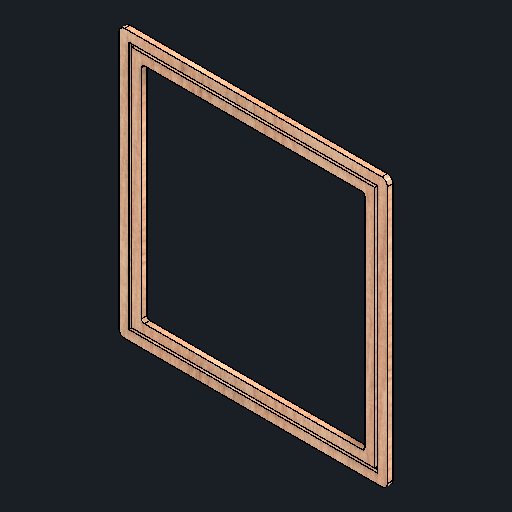
# Autodesk Inventor part: Part1
Saved by Autodesk Inventor 2026.2 (Build 302298000, 298)
## iProperties
Created: 2026-06-15
Part Number: Part1
Material: Wood (Birch)
Document SubType Name: Modeling
Designer: JoshuaEah
Density: 0.55 g/cm^3
Appearance: Birch - Natural Polished
Author: JoshuaEah
Autodesk Inventor part; units mm, degrees
ref_plane "YZ Plane" through (0, 0, 0) normal (1, 0, 0) x (0, 1, 0)
ref_plane "XZ Plane" through (0, 0, 0) normal (0, 1, 0) x (-1, 0, 0)
ref_plane "XY Plane" through (0, 0, 0) normal (0, 0, 1) x (1, 0, 0)
sketch "Sketch1" plane through (0, 0, 0) normal (0, 0, 1) x (1, 0, 0)
  line L0 (0, 0) -> (303.2125, 0)
  line L1 (303.2125, 0) -> (303.2125, 303.2125)
  line L2 (303.2125, 303.2125) -> (0, 303.2125)
  line L3 (0, 303.2125) -> (0, 0)
  line L4 (25.4, 277.8125) -> (277.8125, 277.8125)
  line L5 (277.8125, 277.8125) -> (277.8125, 25.4)
  line L6 (277.8125, 25.4) -> (25.4, 25.4)
  line L7 (25.4, 25.4) -> (25.4, 277.8125)
  line L8 (25.4, 151.6062) -> (277.8125, 151.6063)
  line L9 (151.6062, 277.8125) -> (151.6062, 25.4)
  line L10 (292.1, 292.1) -> (11.1125, 292.1)
  line L11 (11.1125, 292.1) -> (11.1125, 11.1125)
  line L12 (11.1125, 11.1125) -> (292.1, 11.1125)
  line L13 (292.1, 11.1125) -> (292.1, 292.1)
  line L14 (288.925, 288.925) -> (14.2875, 288.925)
  line L15 (14.2875, 288.925) -> (14.2875, 14.2875)
  line L16 (14.2875, 14.2875) -> (288.925, 14.2875)
  line L17 (288.925, 14.2875) -> (288.925, 288.925)
  dimension "d0" = 303.2125
  dimension "d19" = 25.4
  dimension "d20" = 25.4
  dimension "d21" = 25.4
  dimension "d22" = 25.4
  dimension "d37" = 3.175
  dimension "d39" = 11.1125
  dimension "d40" = 11.1125
  constraints: 36 end point, 8 parallel, 5 perpendicular, 4 midpoint, 2 horizontal, 1 coincident, 6 other
  measures "d0" distance of L1.end L2.end
  measures "d19" distance between parallel lines of L3 L7
  measures "d20" distance between parallel lines of L2 L4
  measures "d21" distance between parallel lines of L1 L5
  measures "d22" distance between parallel lines of L0 L6
  measures "d37" distance between parallel lines of L15 L11
  measures "d39" distance between parallel lines of L7 L15
  measures "d40" distance between parallel lines of L11 L3
extrude "Extrusion1" add sketch "Sketch1" against normal blind 6.35 contours L3 L2 L1 L0 | L13 L12 L11 L10 | L17 L16 L15 L14
extrude "Extrusion2" cut sketch "Sketch1" against normal blind 3.175 contours L13 L12 L11 L10
fillet "Fillet1" radius 6.35 4 edges at (0, 303.2125, -3.175) (303.2125, 303.2125, -3.175) (0, 0, -3.175) (303.2125, 0, -3.175)
fillet "Fillet1" radius 3.175 4 edges at (277.8125, 25.4, -3.175) (277.8125, 277.8125, -3.175) (25.4, 277.8125, -3.175) (25.4, 25.4, -3.175)
equation "\"d20\" = d19"
equation "\"d21\" = d19"
equation "\"d22\" = d20"
equation "\"d39\" = d40"
body "Solid1"
